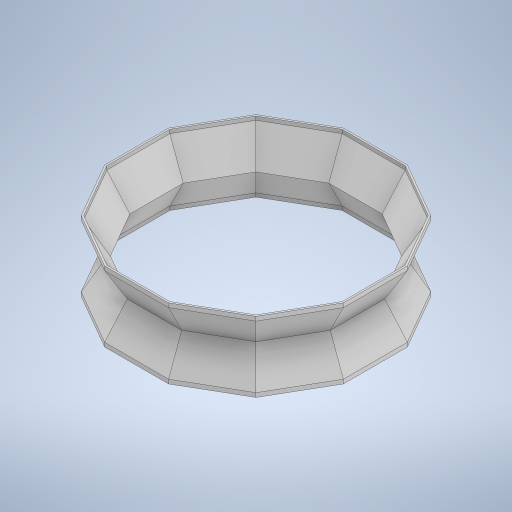
# Autodesk Inventor part: OV-PAM_n_12_standard_1F
Saved by Autodesk Inventor 2024 (Build 280153000, 153)
## iProperties
Created: 2023-08-31
Part Number: OV-PAM_n_12_standard_1F
Material: 일반
Document SubType Name: Modeling
Designer: jsw
Density: 1 g/cm^3
Appearance: 기본값
Author: jsw
Autodesk Inventor part; units mm, degrees
ref_plane "YZ Plane" through (0, 0, 0) normal (1, 0, 0) x (0, 1, 0)
ref_plane "XZ Plane" through (0, 0, 0) normal (0, 1, 0) x (-1, 0, 0)
ref_plane "XY Plane" through (0, 0, 0) normal (0, 0, 1) x (1, 0, 0)
sketch "스케치1" plane through (0, 0, 0) normal (0, 1, 0) x (-1, 0, 0)
  line L0 (-9.1304, 34.075) -> (9.1304, 34.075)
  line L1 (9.1304, 34.075) -> (24.9446, 24.9446)
  line L2 (24.9446, 24.9446) -> (34.075, 9.1304)
  line L3 (34.075, 9.1304) -> (34.075, -9.1304)
  line L4 (34.075, -9.1304) -> (24.9446, -24.9446)
  line L5 (24.9446, -24.9446) -> (9.1304, -34.075)
  line L6 (9.1304, -34.075) -> (-9.1304, -34.075)
  line L7 (-9.1304, -34.075) -> (-24.9446, -24.9446)
  line L8 (-24.9446, -24.9446) -> (-34.075, -9.1304)
  line L9 (-34.075, -9.1304) -> (-34.075, 9.1304)
  line L10 (-34.075, 9.1304) -> (-24.9446, 24.9446)
  line L11 (-24.9446, 24.9446) -> (-9.1304, 34.075)
  line L12 (9.2911, -34.675) -> (-9.2911, -34.675)
  line L13 (-9.2911, -34.675) -> (-25.3838, -25.3838)
  line L14 (-25.3838, -25.3838) -> (-34.675, -9.2911)
  line L15 (-34.675, -9.2911) -> (-34.675, 9.2911)
  line L16 (-34.675, 9.2911) -> (-25.3838, 25.3838)
  line L17 (-25.3838, 25.3838) -> (-9.2911, 34.675)
  line L18 (-9.2911, 34.675) -> (9.2911, 34.675)
  line L19 (9.2911, 34.675) -> (25.3838, 25.3838)
  line L20 (25.3838, 25.3838) -> (34.675, 9.2911)
  line L21 (34.675, 9.2911) -> (34.675, -9.2911)
  line L22 (34.675, -9.2911) -> (25.3838, -25.3838)
  line L23 (25.3838, -25.3838) -> (9.2911, -34.675)
  point P0 (0, 0)
  point P1 (0, 0)
  point P2 (0, 0)
  dimension "d1" = 70.554
  dimension "d2" = 0.6
  constraints: 48 end point, 2 coincident, 2 horizontal, 50 other
  measures "d1" distance of L8.end L2.end
  measures "d2" distance between parallel lines of L3 L21
extrude "돌출1" add sketch "스케치1" along normal blind 9 contours L0 L1 L2 L3 L4 L5 L6 L7 L8 L9 L10 L11 | L12 L13 L14 L15 L16 L17 L18 L19 L20 L21 L22 L23
ref_plane "작업 평면1" through (25.3838, 0, 25.3838) normal (-0.75, -0.5, -0.4330127) x (0.5, 0, -0.8660254)
sketch "스케치2" plane through (34.675, 0, 9.2911) normal (0.8660254, 0, 0.5) x (0.5, 0, -0.8660254)
  line L0 (-18.5823, 0) -> (0, 0) projected
  line L1 (0, 0) -> (0, 9) projected
  line L2 (-18.5823, 9) -> (0, 9) projected
  line L3 (-18.5823, 0) -> (-18.5823, 9) projected
  line L4 (-18.5823, 0) -> (-34.675, 0) projected
  line L5 (-18.5823, 0) -> (-34.1707, 9)
  line L6 (-18.5823, 9) -> (-34.675, 9) projected
  line L7 (0, 0) -> (-1, 9)
  line L8 (-18.5823, 9) -> (-34.1707, 9)
  point P0 (-9.2911, 0)
  point P1 (-34.675, 12)
  dimension "d6" = 150
  dimension "d7" = 1
  constraints: 6 end point, 2 point on line, 1 collinear
  measures "d6" angle of L5 L0
  measures "d7" distance of L1.end L7.end
extrude "돌출2" cut sketch "스케치2" against normal up to surface surface through (25.3838, 0, 25.3838) normal (-0.75, -0.5, -0.4330127)
pattern_circular "원형 패턴1" count 12 over 360 about axis through (0, -10, 0) along (0, 1, 0) of "돌출2"
sketch "스케치3" plane through (0, 0, 0) normal (0, -1, 0) x (1, 0, 0)
  line L0 (-25.3838, -25.3838) -> (-34.675, -9.2911) projected
  line L1 (-9.2911, -34.675) -> (-25.3838, -25.3838) projected
  line L2 (9.2911, -34.675) -> (-9.2911, -34.675) projected
  line L3 (25.3838, -25.3838) -> (9.2911, -34.675) projected
  line L4 (34.675, -9.2911) -> (25.3838, -25.3838) projected
  line L5 (34.675, 9.2911) -> (34.675, -9.2911) projected
  line L6 (25.3838, 25.3838) -> (34.675, 9.2911) projected
  line L7 (9.2911, 34.675) -> (25.3838, 25.3838) projected
  line L8 (-9.2911, 34.675) -> (9.2911, 34.675) projected
  line L9 (-25.3838, 25.3838) -> (-9.2911, 34.675) projected
  line L10 (-34.675, 9.2911) -> (-25.3838, 25.3838) projected
  line L11 (-34.675, -9.2911) -> (-34.675, 9.2911) projected
  point P0 (0, 0)
extrude "돌출3" add sketch "스케치3" along normal blind 1.2
ref_plane "작업 평면2" through (0, 9, 0) normal (0, 1, 0) x (1, 0, 0)
mirror "미러1" about plane through (0, 9, 0) normal (0, 1, 0) of "돌출2", "원형 패턴1", "돌출3", "돌출1"
shell "쉘1" thickness 0.5 removed faces 2 at (8.4613, 19.2, 2.2672) at (8.4613, -1.2, 2.2672)
